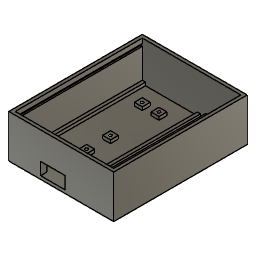
LoRa Base Case (Autodesk Fusion 360 design; units mm, degrees)
Autodesk Fusion 360 part; units mm, degrees
sketch "Skizze1" plane through (0, 0, 0) normal (0, 0, 1) x (1, 0, 0)
  line L0 (0, 0) -> (62, 0)
  line L1 (62, 0) -> (62, -80)
  line L2 (62, -80) -> (0, -80)
  line L3 (0, -80) -> (0, 0)
  line L4 (64, -82) -> (-2, -82)
  line L5 (-2, -82) -> (-2, 2)
  line L6 (-2, 2) -> (64, 2)
  line L7 (64, 2) -> (64, -82)
  line L8 (41, -79) -> (62, -79)
  line L9 (41, -80) -> (41, 0)
  line L10 (40, 0) -> (40, -80)
  line L11 (14.5, -14.5) -> (9.5, -14.5)
  line L12 (9.5, -14.5) -> (9.5, -9.5)
  line L13 (9.5, -9.5) -> (14.5, -9.5)
  line L14 (14.5, -9.5) -> (14.5, -14.5)
  line L15 (14.5, -14.5) -> (9.5, -9.5) construction
  line L16 (9.5, -14.5) -> (14.5, -9.5) construction
  line L17 (25, -14.5) -> (20, -14.5)
  line L18 (20, -14.5) -> (20, -9.5)
  line L19 (20, -9.5) -> (25, -9.5)
  line L20 (25, -9.5) -> (25, -14.5)
  line L21 (25, -14.5) -> (20, -9.5) construction
  line L22 (20, -14.5) -> (25, -9.5) construction
  line L23 (22.5, -42.5) -> (17.5, -42.5)
  line L24 (17.5, -42.5) -> (17.5, -37.5)
  line L25 (17.5, -37.5) -> (22.5, -37.5)
  line L26 (22.5, -37.5) -> (22.5, -42.5)
  line L27 (22.5, -42.5) -> (17.5, -37.5) construction
  line L28 (17.5, -42.5) -> (22.5, -37.5) construction
  line L29 (22.5, -57.5) -> (17.5, -57.5)
  line L30 (17.5, -57.5) -> (17.5, -52.5)
  line L31 (17.5, -52.5) -> (22.5, -52.5)
  line L32 (22.5, -52.5) -> (22.5, -57.5)
  line L33 (22.5, -57.5) -> (17.5, -52.5) construction
  line L34 (17.5, -57.5) -> (22.5, -52.5) construction
  line L35 (-2, -82) -> (64, -82)
  line L36 (64, -82) -> (64, 2)
  line L37 (64, 2) -> (-2, 2)
  line L38 (-2, 2) -> (-2, -82)
  circle A0 centre (12, -12) radius 0.9
  circle A1 centre (22.5, -12) radius 0.9
  circle A2 centre (20, -40) radius 0.9
  circle A3 centre (20, -55) radius 0.9
  point P0 (12, -12)
  point P1 (22.5, -12)
  point P2 (20, -40)
  point P3 (20, -55)
  dimension "d1" = 62
  dimension "d2" = 80
  dimension "d3" = -2
  dimension "d6" = 79
  dimension "d7" = 21
  dimension "d8" = 1
  dimension "d9" = 5
  dimension "d10" = 5
  dimension "d11" = 12
  dimension "d12" = 12
  dimension "d13" = 5
  dimension "d14" = 5
  dimension "d15" = 12
  dimension "d16" = 10.5
  dimension "d17" = 5
  dimension "d18" = 5
  dimension "d19" = 20
  dimension "d20" = 40
  dimension "d21" = 5
  dimension "d22" = 5
  dimension "d23" = 20
  dimension "d24" = 15
  dimension "d44" = 1.8
  dimension "d45" = 1.8
  dimension "d46" = 1.8
  dimension "d47" = 1.8
  constraint horizontal L0
  constraint vertical L1
  constraint horizontal L2
  constraint vertical L3
  constraint coincident L0.start L3.end
  constraint coincident L1 L8.end
  constraint perpendicular L1 L8
  constraint coincident L2 L9.start
  constraint coincident L0 L9.end
  constraint perpendicular L0 L9
  constraint coincident L0 L10.start
  constraint coincident L2 L10.end
  constraint perpendicular L2 L10
  constraint perpendicular L11 L12
  constraint parallel L11 L13
  constraint parallel L12 L14
  constraint horizontal L11
  constraint coincident L15 P0
  constraint coincident L16 P0
  constraint perpendicular L17 L18
  constraint parallel L17 L19
  constraint parallel L18 L20
  constraint horizontal L17
  constraint coincident L21 P1
  constraint coincident L22 P1
  constraint perpendicular L23 L24
  constraint parallel L23 L25
  constraint parallel L24 L26
  constraint horizontal L23
  constraint coincident L27 P2
  constraint coincident L28 P2
  constraint perpendicular L29 L30
  constraint parallel L29 L31
  constraint parallel L30 L32
  constraint horizontal L29
  constraint coincident L33 P3
  constraint coincident L34 P3
  constraint horizontal L35
  constraint vertical L36
  constraint horizontal L37
  constraint vertical L38
  constraint coincident L8.start L9
  constraint coincident P0 A0.centre
  constraint coincident P1 A1.centre
  constraint coincident P2 A2.centre
  constraint coincident P3 A3.centre
  measures "d1" distance of L0.start L0.end
  measures "d2" distance of L0.end L1.end
  measures "d6" distance of L0 L8
  measures "d7" distance of L1 L9
  measures "d8" distance of L9 L10
  measures "d9" distance of L11.start L11.end
  measures "d10" distance of L11.start L13.end
  measures "d11" distance of L3 P0
  measures "d12" distance of L0 P0
  measures "d13" distance of L17.start L17.end
  measures "d14" distance of L17.start L19.end
  measures "d15" distance of L0 P1
  measures "d16" distance of P0 P1
  measures "d17" distance of L23.start L23.end
  measures "d18" distance of L23.start L25.end
  measures "d19" distance of L3 P2
  measures "d20" distance of L0 P2 L3.end
  measures "d21" distance of L29.start L29.end
  measures "d22" distance of L29.start L31.end
  measures "d23" distance of L3 P3
  measures "d24" distance of P2 P3
  measures "d44" diameter of A0
  measures "d45" diameter of A1
  measures "d46" diameter of A2
  measures "d47" diameter of A3
extrude "Extrusion2" add sketch "Skizze1" along normal blind 25 contours L4 L5 L6 L7 L35 L36 L37 L38 makes body 1
extrude "Extrusion3" add sketch "Skizze1" along normal blind 2 separate body contours L11 L12 L13 L14 | L17 L18 L19 L20 | L23 L24 L25 L26 | L29 L30 L31 L32 makes body 2 at (19.9776, -41.9658, 0) makes body 3 at (22.5224, -10.0342, 0) makes body 4 at (20.0224, -56.9658, 0) makes body 5 at (11.9776, -10.0342, 0)
extrude "Extrusion4" add sketch "Skizze1" along normal blind 4 contours L0 L2 L9 L10 | L1 L2 L8 L9 bodies 1
extrude "Extrusion6" add sketch "Skizze1" against normal blind 2 separate body contours L0 L2 L3 L10 | L0 L2 L9 L10 | L0 L1 L8 L9 | L1 L2 L8 L9 | L4 L5 L6 L7 L35 L36 L37 L38 | L11 L12 L13 L14 | L17 L18 L19 L20 | L23 L24 L25 L26 | L29 L30 L31 L32 | A0 | A1 | A2 | A3 makes body 6
sketch "Skizze2" plane through (0, 0, 0) normal (0, 0, 1) x (-1, 0, 0)
  line L0 (2, -2) -> (2, 82)
  line L1 (2, 82) -> (-64, 82)
  line L2 (-64, 82) -> (-64, -2)
  line L3 (-64, -2) -> (2, -2)
  line L4 (0, 0) -> (-2, 0)
  line L5 (-2, 0) -> (-2, 66)
  line L6 (-2, 66) -> (0, 66)
  line L7 (0, 66) -> (0, 0)
  line L8 (-34.6, 0) -> (-36.6, 0)
  line L9 (-36.6, 0) -> (-36.6, 66)
  line L10 (-36.6, 66) -> (-34.6, 66)
  line L11 (-34.6, 66) -> (-34.6, 0)
  dimension "d37" = 66
  dimension "d38" = 2
  dimension "d39" = 66
  dimension "d40" = 36.6
  dimension "d41" = 2
  constraint horizontal L4
  constraint vertical L5
  constraint horizontal L6
  constraint vertical L7
  constraint coincident L4.start L7.end
  constraint horizontal L8
  constraint vertical L9
  constraint horizontal L10
  constraint vertical L11
  measures "d37" distance of L4.end L5.end
  measures "d38" distance of L5.end L6.end
  measures "d39" distance of L8.end L9.end
  measures "d40" distance of L7 L9
  measures "d41" distance of L9.end L10.end
extrude "Extrusion7" add sketch "Skizze2" along normal blind 2 contours L4 L5 L6 L7 | L8 L9 L10 L11 bodies 1 6
sketch "Skizze4" plane through (0, -82, 0) normal (0, -1, 0) x (1, 0, 0)
  line L0 (64, -2) -> (64, 25)
  line L1 (64, 25) -> (-2, 25)
  line L2 (-2, 25) -> (-2, -2)
  line L3 (-2, -2) -> (64, -2)
  line L4 (18, 7.8) -> (33.4, 7.8)
  line L5 (33.4, 7.8) -> (33.4, 0)
  line L6 (33.4, 0) -> (18, 0)
  line L7 (18, 0) -> (18, 7.8)
  dimension "d53" = 15.4
  dimension "d54" = 7.8
  dimension "d55" = 20
  dimension "d56" = 2
  constraint horizontal L4
  constraint vertical L5
  constraint horizontal L6
  constraint vertical L7
  measures "d53" distance of L4.start L4.end
  measures "d54" distance of L4.end L5.end
  measures "d55" distance of L2 L7
  measures "d56" distance of L3 L6
extrude "Extrusion9" cut sketch "Skizze4" against normal up to surface (2 mm away) contours L4 L5 L6 L7 bodies 1
sketch "Skizze5" plane through (0, -80, 0) normal (0, 1, 0) x (-1, 0, 0)
  line L0 (-33.4, 0) -> (-33.4, 7.8)
  line L1 (-33.4, 7.8) -> (-18, 7.8)
  line L2 (-18, 7.8) -> (-18, 0)
  line L3 (-18, 0) -> (0, 0)
  line L4 (0, 0) -> (0, 25)
  line L5 (0, 25) -> (-62, 25)
  line L6 (-62, 25) -> (-62, 4)
  line L7 (-62, 4) -> (-40, 4)
  line L8 (-40, 4) -> (-40, 0)
  line L9 (-40, 0) -> (-33.4, 0)
  line L10 (-34.4, 0) -> (-34.4, 8.8)
  line L11 (-34.4, 8.8) -> (-17, 8.8)
  line L12 (-17, 8.8) -> (-17, 0)
  dimension "d59" = -1
extrude "Extrusion10" add sketch "Skizze5" along normal blind 2 contours L0 L1 L2 L3 L9 L10 L11 L12 bodies 1
sketch "Skizze6" plane through (62, 0, 0) normal (-1, 0, 0) x (0, -1, 0)
  line L0 (79, 0) -> (79, 4)
  line L1 (79, 4) -> (80, 4)
  line L2 (80, 4) -> (80, 25)
  line L3 (80, 25) -> (0, 25)
  line L4 (0, 25) -> (0, 0)
  line L5 (0, 0) -> (79, 0)
  line L6 (0, 22) -> (80, 22)
  line L7 (80, 22) -> (80, 20.5)
  line L8 (80, 20.5) -> (0, 20.5)
  line L9 (0, 20.5) -> (0, 22)
  dimension "d62" = 1.5
  dimension "d63" = 3
  constraint horizontal L6
  constraint vertical L7
  constraint horizontal L8
  constraint vertical L9
  constraint coincident L2 L7.end
  constraint coincident L4 L6.start
  measures "d62" distance of L6 L8
  measures "d63" distance of L3 L6
extrude "Extrusion11" cut sketch "Skizze6" against normal blind 1 contours L2 L4 L6 L7 L8 L9 bodies 1
sketch "Skizze7" plane through (0, 0, 0) normal (1, 0, 0) x (0, 1, 0)
  line L0 (-66, 0) -> (-66, 2)
  line L1 (-66, 2) -> (0, 2)
  line L2 (0, 2) -> (0, 25)
  line L3 (0, 25) -> (-80, 25)
  line L4 (-80, 25) -> (-80, 0)
  line L5 (-80, 0) -> (-66, 0)
  line L6 (0, 22) -> (-80, 22)
  line L7 (-80, 22) -> (-80, 20.5)
  line L8 (-80, 20.5) -> (0, 20.5)
  line L9 (0, 20.5) -> (0, 22)
  dimension "d66" = 1.5
  dimension "d67" = 3
  constraint horizontal L6
  constraint vertical L7
  constraint horizontal L8
  constraint vertical L9
  constraint coincident L4 L7.end
  constraint coincident L2 L6.start
  measures "d66" distance of L6 L8
  measures "d67" distance of L3 L6
extrude "Extrusion12" cut sketch "Skizze7" against normal blind 1 contours L2 L4 L6 L7 L8 L9 bodies 1
